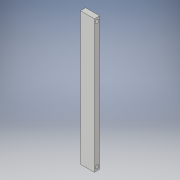
# Autodesk Inventor part: ArmProto
Saved by Autodesk Inventor 2017 (Build 210142000, 142)
## iProperties
Created: 2017-09-30
Part Number: ArmProto
Material: Generic
Document SubType Name: Modeling
Designer: User
Density: 1 g/cm^3
Appearance: Default
Author: User
Autodesk Inventor part; units mm, degrees
ref_plane "YZ Plane" through (0, 0, 0) normal (1, 0, 0) x (0, 1, 0)
ref_plane "XZ Plane" through (0, 0, 0) normal (0, 1, 0) x (-1, 0, 0)
ref_plane "XY Plane" through (0, 0, 0) normal (0, 0, 1) x (1, 0, 0)
sketch "Sketch1" plane through (0, 0, 0) normal (1, 0, 0) x (0, 1, 0)
  line L0 (0, 0) -> (482.6, 0)
  line L1 (482.6, 0) -> (482.6, -19.05)
  line L2 (482.6, -19.05) -> (0, -19.05)
  line L3 (0, -19.05) -> (0, 0)
  circle A0 centre (469.9, -9.525) radius 6.35
  circle A1 centre (12.7, -9.525) radius 6.35
  dimension "d0" = 482.6
  dimension "d1" = 19.05
  dimension "d2" = 12.7
  dimension "d3" = 12.7
  dimension "d4" = 12.7
  dimension "d5" = 12.7
  constraints: 8 end point, 2 centre point, 2 parallel, 1 horizontal, 1 perpendicular
  measures "d0" distance of L1.end L2.end
  measures "d1" distance of L0.end L1.end
  measures "d2" diameter of A0
  measures "d3" diameter of A1
  measures "d4" distance from line of L3 A1.centre
  measures "d5" distance from line of L1 A0.centre
extrude "Extrusion1" add sketch "Sketch1" along normal blind 50.8
equation "\"d5\" = d4"
body "Solid1"
